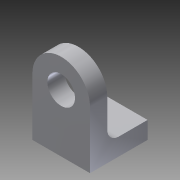
# Autodesk Inventor part: support_electronics
Saved by Autodesk Inventor 2015 (Build 190159000, 159)
## iProperties
Created: 2016-05-30
Part Number: support_electronics
Material: Plástico ABS
Document SubType Name: Modeling
Designer: JavierPC
Density: 1.06 g/cm^3
Appearance: Suave - Blanco
Author: JavierPC
Autodesk Inventor part; units mm, degrees
ref_plane "YZ Plane" through (0, 0, 0) normal (1, 0, 0) x (0, 1, 0)
ref_plane "XZ Plane" through (0, 0, 0) normal (0, 1, 0) x (-1, 0, 0)
ref_plane "XY Plane" through (0, 0, 0) normal (0, 0, 1) x (1, 0, 0)
sketch "Boceto2" plane through (0, 0, 0) normal (0, 1, 0) x (-1, 0, 0)
  line L0 (2.5, 5) -> (2.5, 0)
  line L1 (2.5, 0) -> (-2.5, 0)
  line L2 (-2.5, 0) -> (-2.5, 5)
  arc A0 (2.5, 5) -> (-2.5, 5) centre (0, 5) ccw
  circle A1 centre (0, 5) radius 1.2
  point P0 (0, 0)
  point P1 (0, 0)
  dimension "d2" = 5
  dimension "d3" = 5
  dimension "d4" = 2.4
  constraints: 6 end point, 2 centre point, 2 coincident, 2 point on circle, 1 midpoint, 1 parallel
  measures "d2" distance of L0.end L1.end
  measures "d3" distance of L0.start L0.end
  measures "d4" diameter of A1
extrude "Extrusión1" add sketch "Boceto2" along normal blind 1.5
sketch "Boceto3" plane through (0, 0, 0) normal (0, 1, 0) x (-1, 0, 0)
  line L0 (-2.5, 1.5) -> (2.5, 1.5)
  line L1 (2.5, 1.5) -> (2.5, 0)
  line L2 (2.5, 0) -> (-2.5, 0)
  line L3 (-2.5, 0) -> (-2.5, 1.5)
  line L4 (-2.5, 0) -> (2.5, 0) projected
  point P0 (0, 0)
  point P1 (0, 0)
  dimension "d7" = 5
  dimension "d8" = 1.5
  constraints: 8 end point, 2 midpoint, 2 parallel, 1 horizontal, 1 perpendicular
  measures "d7" distance of L1.end L2.end
  measures "d8" distance of L0.end L1.end
extrude "Extrusión2" add sketch "Boceto3" along normal blind 5
fillet "Empalme1" radius 1 1 edges at (0, 1.5, 1.5)
